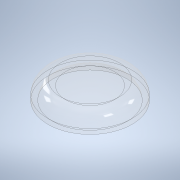
# Autodesk Inventor part: camera cover
Saved by Autodesk Inventor 2022.2 (Build 262287000, 287)
## iProperties
Created: 2022-02-22
Part Number: camera cover
Material: PET Plastic
Document SubType Name: Modeling
Designer: ONG
Density: 1.541 g/cm^3
Appearance: Polycarbonate - Clear
Author: ONG
Autodesk Inventor part; units mm, degrees
ref_plane "YZ Plane" through (0, 0, 0) normal (1, 0, 0) x (0, 1, 0)
ref_plane "XZ Plane" through (0, 0, 0) normal (0, 1, 0) x (-1, 0, 0)
ref_plane "XY Plane" through (0, 0, 0) normal (0, 0, 1) x (1, 0, 0)
sketch "Sketch2" plane through (0, 0, 0) normal (1, 0, 0) x (0, 1, 0)
  line L0 (0, 0) -> (5, 0)
  line L1 (5, 0) -> (5, 9.7075)
  line L2 (0, 14.7075) -> (0, 14.7075)
  arc A0 (5, 9.7075) -> (0, 14.7075) centre (0, 9.7075) ccw
  line L3 (5, 0) -> (7, 0)
  line L4 (2, 16.7075) -> (0, 16.7075)
  line L5 (0, 16.7075) -> (0, 14.7075)
  line L6 (7, 11.7075) -> (7, 0)
  arc A1 (7, 11.7075) -> (2, 16.7075) centre (2, 11.7075) ccw
  dimension "d1" = 5
  dimension "d2" = 5
  dimension "d3" = 2
  dimension "d5" = 5
  constraints: 14 end point, 4 point on circle, 4 tangent, 3 horizontal, 2 centre point, 2 perpendicular, 1 vertical
  measures "d1" distance of L0.start L0.end
  measures "d2" radius of A0
  measures "d3" distance of L0.end L3.end
  measures "d5" radius of A1
revolve "Revolution1" add sketch "Sketch2" angle 360 about axis through (0, 0, 0) along (0, 1, 0)
body "Solid1"
